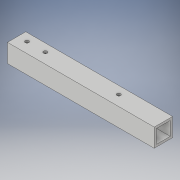
# Autodesk Inventor part: Tube Beam
Saved by Autodesk Inventor 2018 (Build 220112000, 112)
## iProperties
Created: 2018-12-06
Part Number: Tube Beam
Material: Generic
Document SubType Name: Modeling
Designer: gbgic
Density: 1 g/cm^3
Appearance: Default
Author: gbgic
Autodesk Inventor part; units mm, degrees
ref_plane "YZ Plane" through (0, 0, 0) normal (1, 0, 0) x (0, 1, 0)
ref_plane "XZ Plane" through (0, 0, 0) normal (0, 1, 0) x (-1, 0, 0)
ref_plane "XY Plane" through (0, 0, 0) normal (0, 0, 1) x (1, 0, 0)
sketch "Sketch1" plane through (0, 0, 0) normal (1, 0, 0) x (0, 1, 0)
  line L0 (6.0697, 14.4062) -> (-19.3303, 14.4062)
  line L1 (-19.3303, 14.4062) -> (-19.3303, -10.9938)
  line L2 (-19.3303, -10.9938) -> (6.0697, -10.9938)
  line L3 (6.0697, -10.9938) -> (6.0697, 14.4062)
  line L4 (2.8947, 11.2312) -> (-16.1553, 11.2312)
  line L5 (-16.1553, 11.2312) -> (-16.1553, -7.8188)
  line L6 (-16.1553, -7.8188) -> (2.8947, -7.8188)
  line L7 (2.8947, -7.8188) -> (2.8947, 11.2312)
  point P0 (0, 0)
  dimension "d0" = 25.4
  dimension "d1" = 25.4
  dimension "d2" = 3.175
  constraints: 16 end point, 4 parallel, 2 perpendicular, 1 horizontal, 3 other
  measures "d0" distance of L2.end L1.end
  measures "d1" distance of L1.end L0.end
  measures "d2" distance between parallel lines of L3 L7
extrude "Extrusion1" add sketch "Sketch1" along normal blind 304.8
sketch "Sketch2" plane through (0, 6.0697, 14.4062) normal (0, 1, 0) x (1, 0, 0)
  line L0 (0, 14.4062) -> (12.7, 14.4062)
  line L1 (12.7, 14.4062) -> (38.1, 14.4062)
  circle A0 centre (12.7, 14.4062) radius 2.5797
  circle A1 centre (38.1, 14.4062) radius 2.5797
  line L2 (304.8, 22.225) -> (304.8, 3.175) projected
  circle A2 centre (139.7096, 14.4062) radius 2.5797
  dimension "d5" = 12.7
  dimension "d6" = 25.4
  dimension "d7" = 5.1594
  dimension "d8" = 5.1594
  dimension "d13" = 5.1594
  constraints: 4 end point, 3 centre point, 2 coincident, 1 horizontal, 1 point on line
  measures "d5" distance of L0.start L0.end
  measures "d6" distance of L0.end L1.end
  measures "d7" diameter of A0
  measures "d8" diameter of A1
  measures "d13" diameter of A2
extrude "Extrusion3" cut sketch "Sketch2" against normal blind 304.8
sketch "Sketch3" plane through (0, 6.0697, 14.4062) normal (0, 1, 0) x (1, 0, 0)
  line L0 (304.8, 3.175) -> (304.8, 22.225) projected
  line L1 (304.8, 12.7) -> (203.2, 12.7)
  line L2 (0, 25.4) -> (304.8, 25.4) projected
  line L3 (0, 0) -> (304.8, 0) projected
  line L4 (203.2, 25.4) -> (304.8, 25.4)
  line L5 (304.8, 25.4) -> (304.8, 0)
  line L6 (304.8, 0) -> (203.2, 0)
  line L7 (203.2, 0) -> (203.2, 25.4)
  point P0 (0, 14.4062)
  dimension "d18" = 101.6
  constraints: 10 end point, 2 horizontal, 2 parallel, 1 midpoint, 1 perpendicular, 1 point on line
  measures "d18" distance of L1.start L1.end
extrude "Extrusion4" cut sketch "Sketch3" against normal blind 304.8
body "Solid1"
